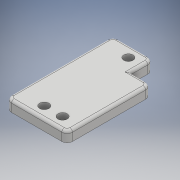
# Autodesk Inventor part: SyringeServoBaseClamp
Saved by Autodesk Inventor 2018 (Build 220112000, 112)
## iProperties
Created: 2018-05-20
Part Number: SyringeServoBaseClamp
Material: Generic
Document SubType Name: Modeling
Designer: reide
Density: 1 g/cm^3
Appearance: Default
Author: reide
Autodesk Inventor part; units mm, degrees
ref_plane "YZ Plane" through (0, 0, 0) normal (1, 0, 0) x (0, 1, 0)
ref_plane "XZ Plane" through (0, 0, 0) normal (0, 1, 0) x (-1, 0, 0)
ref_plane "Work Plane1" through (-7.86, -16.002, 12.7) normal (0, 0, 1) x (1, 0, 0)
sketch "Sketch5" plane through (0, 0, 0) normal (0, 0, 1) x (1, 0, 0)
  line L0 (7.248, 20) -> (7.248, 11.68) projected
  line L1 (-5.86, 20) -> (7.248, 20) projected
  arc A0 (-5.86, 20) -> (-7.86, 18) centre (-5.86, 18) ccw projected
  line L2 (-7.86, 11.68) -> (-7.86, 18) projected
  line L3 (-3.792, 11.68) -> (-7.86, 11.68) projected
  line L4 (-3.792, 16.252) -> (-3.792, 11.68) projected
  line L5 (-0.752, 16.252) -> (-3.792, 16.252) projected
  line L6 (-0.752, 11.68) -> (-0.752, 16.252) projected
  line L7 (7.248, 11.68) -> (-0.752, 11.68) projected
  arc A1 (-7.86, -18) -> (-5.86, -20) centre (-5.86, -18) ccw projected
  line L8 (13, -20) -> (-5.86, -20) projected
  arc A2 (13, -20) -> (15, -18) centre (13, -18) ccw projected
  line L9 (15, -11.68) -> (15, -18) projected
  line L10 (-0.752, -11.68) -> (15, -11.68) projected
  line L11 (-0.752, -16.252) -> (-0.752, -11.68) projected
  line L12 (-3.792, -16.252) -> (-0.752, -16.252) projected
  line L13 (-3.792, -11.68) -> (-3.792, -16.252) projected
  line L14 (-7.86, -11.68) -> (-3.792, -11.68) projected
  line L15 (-7.86, -18) -> (-7.86, -11.68) projected
  line L16 (-0.752, 16.252) -> (-3.792, 16.252)
  line L17 (-3.792, 16.252) -> (-3.792, -16.252)
  line L18 (-3.792, -16.252) -> (-0.752, -16.252)
  line L19 (-0.752, -16.252) -> (-0.752, 16.252)
  line L20 (7.248, 11.68) -> (-7.86, 11.68)
  line L21 (-7.86, 11.68) -> (-7.86, -11.68)
  line L22 (-7.86, -11.68) -> (7.248, -11.68)
  line L23 (7.248, -11.68) -> (7.248, 11.68)
  line L24 (15, 11.43) -> (-1.002, 11.43) projected
  line L25 (15, 11.43) -> (7.248, 11.43)
  line L26 (7.248, 11.43) -> (7.248, -11.68)
  line L27 (7.248, -11.68) -> (15, -11.68)
  line L28 (15, -11.68) -> (15, 11.43)
  point P0 (0, 0)
  constraints: 24 end point, 6 parallel, 3 horizontal, 3 perpendicular
extrude "Extrusion3" add sketch "Sketch5" along normal blind 4
sketch "Sketch6" plane through (0, 0, 4) normal (0, 0, 1) x (1, 0, 0)
  line L0 (7.248, 11.43) -> (7.248, 20) projected
  line L1 (7.248, 15.715) -> (2.248, 15.715)
  circle A0 centre (2.248, 15.715) radius 1.75
  line L2 (14.9228, 0) -> (0, 0)
  line L3 (7.248, 20) -> (7.248, 15.715)
  line L4 (15, -18) -> (15, 11.43) projected
  line L5 (15, -20) -> (15, -15.715)
  line L6 (15, -15.715) -> (-7.86, -15.715)
  line L7 (-7.86, 18) -> (-7.86, -18) projected
  line L8 (15, -15.715) -> (9, -15.715)
  circle A1 centre (9, -15.715) radius 1.75
  line L9 (-7.86, -15.715) -> (2.14, -15.715)
  circle A2 centre (2.14, -15.715) radius 1.75
  dimension "d14" = 5
  dimension "d15" = 3.5
  dimension "d16" = 4.285
  dimension "d17" = 6
  dimension "d18" = 3.5
  dimension "d19" = 10
  dimension "d20" = 3.5
  constraints: 14 end point, 4 point on line, 3 centre point, 3 coincident, 2 horizontal, 1 midpoint, 1 parallel, 1 perpendicular
  measures "d14" distance of L1.start L1.end
  measures "d15" diameter of A0
  measures "d16" distance of L5.start L5.end
  measures "d17" distance of L5.end L8.end
  measures "d18" diameter of A1
  measures "d19" distance of L6.end L9.end
  measures "d20" diameter of A2
extrude "Extrusion4" cut sketch "Sketch6" against normal blind 4
fillet "Fillet1" radius 2 2 edges at (7.248, 20, 2) (15, 11.43, 2)
fillet "Fillet2" radius 1 11 edges at (6.6622, 19.4142, 4) (-0.306, 20, 4) (-7.2742, 19.4142, 4) (-7.86, 0, 4) (-7.2742, -19.4142, 4) (3.57, -20, 4) (14.4142, -19.4142, 4) (15, -4.285, 4) (14.4142, 10.8442, 4) (10.124, 11.43, 4) (7.248, 14.715, 4)
body "Solid2"
